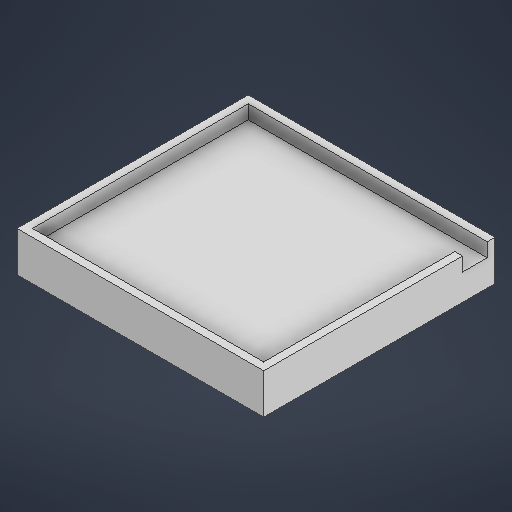
# Autodesk Inventor part: Photosynthetic_Wind_Base
Saved by Autodesk Inventor 2026.1 (Build 301233020, 233B)
## iProperties
Created: 2025-10-22
Part Number: Photosynthetic_Wind_Base
Material: Generic
Document SubType Name: Modeling
Designer: spyro
Density: 1 g/cm^3
Appearance: Default
Author: spyro
Autodesk Inventor part; units mm, degrees
ref_plane "YZ Plane" through (0, 0, 0) normal (1, 0, 0) x (0, 1, 0)
ref_plane "XZ Plane" through (0, 0, 0) normal (0, 1, 0) x (-1, 0, 0)
ref_plane "XY Plane" through (0, 0, 0) normal (0, 0, 1) x (1, 0, 0)
sketch "Sketch1" plane through (0, 0, 0) normal (0, 0, 1) x (1, 0, 0)
  line L0 (0, 0) -> (0, 33.02)
  line L1 (0, 33.02) -> (203.2, 33.02)
  line L2 (203.2, 33.02) -> (203.2, 0)
  line L3 (203.2, 0) -> (0, 0)
  dimension "d0" = 203.2
  dimension "d1" = 33.02
  constraints: 8 end point, 3 perpendicular, 1 vertical
  measures "d0" distance of L0.end L1.end
  measures "d1" distance of L1.end L2.end
extrude "Extrusion1" add sketch "Sketch1" along normal blind 190.5
sketch "Sketch2" plane through (0, 33.02, 0) normal (0, 1, 0) x (1, 0, 0)
  line L0 (196.85, -184.15) -> (6.35, -184.15)
  line L1 (6.35, -184.15) -> (6.35, -6.35)
  line L2 (6.35, -6.35) -> (196.85, -6.35)
  line L3 (196.85, -6.35) -> (196.85, -184.15)
  line L4 (203.2, 0) -> (203.2, -190.5) projected
  line L5 (203.2, 0) -> (0, 0) projected
  line L6 (0, 0) -> (0, -190.5) projected
  dimension "d4" = 190.5
  dimension "d5" = 177.8
  dimension "d6" = 6.35
  dimension "d7" = 6.35
  constraints: 8 end point, 2 perpendicular, 1 horizontal, 1 parallel
  measures "d4" distance of L0.start L0.end
  measures "d5" distance of L2.end L0.start
  measures "d6" distance between parallel lines of L5 L2
  measures "d7" distance between parallel lines of L6 L1
extrude "Extrusion2" cut sketch "Sketch2" against normal blind 11.43
sketch "Sketch3" plane through (203.2, 0, 0) normal (1, 0, 0) x (0, 0, -1)
  line L0 (-6.35, 21.59) -> (-184.15, 21.59) projected
  line L1 (0, 33.02) -> (-190.5, 33.02) projected
  line L2 (-26.7226, 33.02) -> (-26.7226, 21.59)
  line L3 (-6.35, 21.59) -> (-6.35, 33.02)
  line L4 (-26.7226, 33.02) -> (-6.35, 33.02)
  point P0 (0, 0)
  constraints: 6 end point, 3 point on line, 1 collinear, 1 parallel, 1 perpendicular
extrude "Extrusion3" cut sketch "Sketch3" against normal blind 11.43
body "Solid1"
